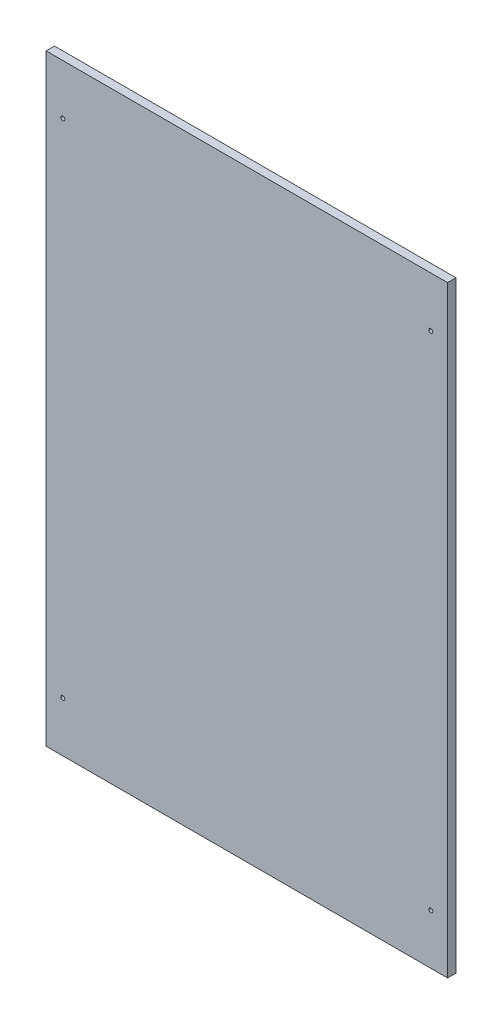
# Autodesk Inventor part: Part7
Saved by Autodesk Inventor 2015 (Build 190159000, 159)
## iProperties
Created: 2015-07-05
Part Number: Part7
Material: Generic
Document SubType Name: Modeling
Designer: tsayman
Density: 1 g/cm^3
Appearance: Default
Author: tsayman
Autodesk Inventor part; units mm, degrees
ref_plane "YZ Plane" through (0, 0, 0) normal (1, 0, 0) x (0, 1, 0)
ref_plane "XZ Plane" through (0, 0, 0) normal (0, 1, 0) x (-1, 0, 0)
ref_plane "XY Plane" through (0, 0, 0) normal (0, 0, 1) x (1, 0, 0)
sketch "Sketch1" plane through (0, 0, 0) normal (0, 0, 1) x (1, 0, 0)
  line L0 (-12.7, -1465.0988) -> (292.1, -1465.0988)
  line L1 (292.1, -1465.0988) -> (292.1, -1922.2988)
  line L2 (292.1, -1922.2988) -> (-12.7, -1922.2988)
  line L3 (-12.7, -1922.2988) -> (-12.7, -1465.0988)
  point P0 (0, 0)
  dimension "d0" = 304.8
  dimension "d1" = 457.2
  constraints: 8 end point, 2 parallel, 1 horizontal, 1 perpendicular
  measures "d0" distance of L1.end L2.end
  measures "d1" distance of L0.end L1.end
extrude "Extrusion1" add sketch "Sketch1" along normal blind 6.35
sketch "Sketch2" plane through (0, 0, 6.35) normal (0, 0, 1) x (1, 0, 0)
  circle A0 centre (0, -1503.1988) radius 1.5875
  circle A1 centre (279.4, -1503.1988) radius 1.5875
  circle A2 centre (0, -1884.1988) radius 1.5875
  circle A3 centre (279.4, -1884.1988) radius 1.5875
  line L0 (292.1, -1922.2988) -> (292.1, -1465.0988) projected
  line L1 (-12.7, -1465.0988) -> (-12.7, -1922.2988) projected
  line L2 (292.1, -1922.2988) -> (-12.7, -1922.2988) projected
  line L3 (292.1, -1465.0988) -> (-12.7, -1465.0988) projected
  point P0 (0, 0)
  dimension "d4" = 3.175
  dimension "d5" = 12.7
  dimension "d6" = 12.7
  dimension "d7" = 38.1
  dimension "d9" = 38.1
  constraints: 4 centre point, 3 equal radius, 2 horizontal alignment, 2 vertical alignment
  measures "d4" diameter of A1
  measures "d5" distance from line of L0 A3.centre
  measures "d6" distance from line of L1 A2.centre
  measures "d7" distance from line of L2 A3.centre
  measures "d9" distance from line of L3 A0.centre
extrude "Extrusion2" cut sketch "Sketch2" against normal blind 25.4 contours A0 | A1 | A2 | A3
body "Solid1"
